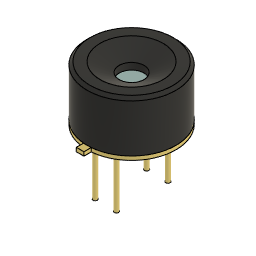
MLX90641 v3 (Autodesk Fusion 360 design; units mm, degrees)
Autodesk Fusion 360 part; units mm, degrees
sketch "Sketch1" plane through (0, 0, 0) normal (0, 0, 1) x (1, 0, 0)
  circle A0 centre (0, 0) radius 4.65
  circle A1 centre (0, 0) radius 1.3
  line L0 (-0.4, -5.4) -> (0.4, -5.4)
  line L1 (0.4, -5.4) -> (0.4, -4.6328)
  line L2 (-0.4, -4.6328) -> (-0.4, -5.4)
  circle A2 centre (-1.1174, -2.6977) radius 0.225
  circle A3 centre (1.1174, -2.6977) radius 0.225
  circle A4 centre (1.1174, 2.6977) radius 0.225
  circle A5 centre (-1.1174, 2.6977) radius 0.225
  dimension "d11" = 360
  constraint coincident A0.centre A1.centre
  constraint horizontal L0
  constraint vertical L1
  constraint vertical L2
  constraint coincident A0 L2.start
  constraint coincident A0 L1.end
extrude "Extrude1" add sketch "Sketch1" along normal blind 5.7 and the other way blind -0.4 contours A0 | A2 | A3 | A4 | A5 makes body 1
extrude "Extrude2" add sketch "Sketch1" along normal blind 0.4 separate body makes body 2
extrude "Extrude3" add sketch "Sketch1" against normal blind 6 separate body contours A2 | A3 | A4 | A5 makes body 3 at (-0.8927, -2.7089, -4) makes body 4 at (-0.8927, 2.6865, -4) makes body 5 at (1.3422, -2.7089, -4) makes body 6 at (1.3422, 2.6865, -4)
extrude "Extrude4" add sketch "Sketch1" along normal blind 4 separate body contours A1 makes body 7
chamfer "Chamfer1" distance 0.3 angle 45 1 edges at (-4.3353, -1.6815, 5.7) on bodies 1
chamfer "Chamfer2" distance 2 distance2 1 1 edges at (-1.212, 0.4701, 5.7) measured on face at (-0.0651, -3.3238, 5.7) on bodies 1
